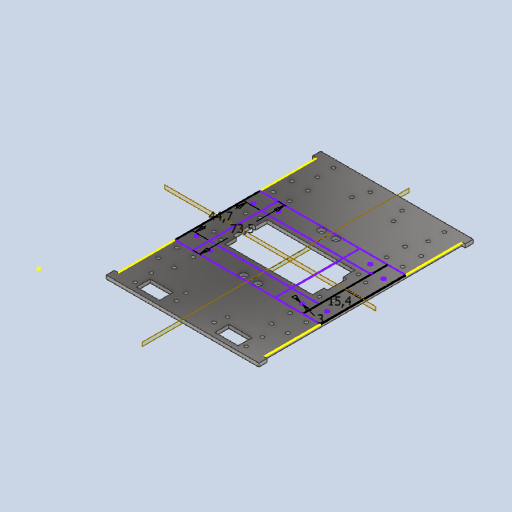
# Autodesk Inventor part: maze_04
Saved by Autodesk Inventor 2022 (Build 260153000, 153)
## iProperties
Created: 2022-07-14
Part Number: maze_04
Material: Сталь нержавеющая, 440C
Document SubType Name: Modeling
Designer: akapu
Density: 7.75 g/cm^3
Appearance: Сталь — полированная
Author: akapu
Autodesk Inventor part; units mm, degrees
ref_plane "YZ Plane" through (0, 0, 0) normal (1, 0, 0) x (0, 1, 0)
ref_plane "XZ Plane" through (0, 0, 0) normal (0, 1, 0) x (-1, 0, 0)
ref_plane "XY Plane" through (0, 0, 0) normal (0, 0, 1) x (1, 0, 0)
sketch "Эскиз2" plane through (0, 0, 0) normal (0, 1, 0) x (-1, 0, 0)
  line L0 (-37, -102) -> (-37, -192)
  line L1 (-166, -192) -> (-163, -192)
  line L2 (-163, -192) -> (-163, -102)
  line L3 (-37, -192) -> (-34, -192)
  line L4 (-34, -200) -> (-166, -200)
  line L5 (-37, -98) -> (-37, -102)
  line L6 (-163, -98) -> (-163, -102)
  line L7 (-166, -192) -> (-166, -200)
  line L8 (-34, -192) -> (-34, -200)
  line L9 (-163, -192) -> (-163, -157)
  line L10 (-163, -157) -> (-37, -157)
  line L11 (-163, -157) -> (-163, -63)
  line L12 (-163, -63) -> (-37, -63)
  line L13 (-34, -34.5) -> (-166, -34.5)
  line L14 (-166, -34.5) -> (-163, -34.5)
  line L15 (-163, -42.5) -> (-166, -42.5)
  line L16 (-166, -42.5) -> (-166, -34.5)
  line L17 (-34, -34.5) -> (-37, -34.5)
  line L18 (-37, -42.5) -> (-34, -42.5)
  line L19 (-37, -98) -> (-37, -34.5)
  line L20 (-34, -34.5) -> (-34, -42.5)
  line L21 (-163, -63) -> (-163, -34.5)
  line L22 (-34, -34.5) -> (-166, -34.5)
  line L23 (-166, -34.5) -> (-166, -24.5)
  line L24 (-166, -24.5) -> (-34, -24.5)
  line L25 (-34, -24.5) -> (-34, -34.5)
  line L26 (-166, -24.5) -> (-34, -24.5)
  line L27 (-34, -24.5) -> (-34, -32.5)
  line L28 (-34, -32.5) -> (-166, -32.5)
  line L29 (-166, -32.5) -> (-166, -24.5)
  line L30 (-34, -32.5) -> (-37, -32.5)
  line L31 (-37, -32.5) -> (-37, -42.5)
  line L32 (-37, -42.5) -> (-34, -42.5)
  line L33 (-34, -42.5) -> (-34, -32.5)
  line L34 (-166, -32.5) -> (-163, -32.5)
  line L35 (-163, -32.5) -> (-163, -42.5)
  line L36 (-163, -42.5) -> (-166, -42.5)
  line L37 (-166, -42.5) -> (-166, -32.5)
  line L38 (-166, -200) -> (-34, -200)
  line L39 (-34, -200) -> (-34, -210)
  line L40 (-34, -210) -> (-166, -210)
  line L41 (-166, -210) -> (-166, -200)
  line L42 (-34, -210) -> (-166, -210)
  line L43 (-166, -210) -> (-166, -202)
  line L44 (-166, -202) -> (-34, -202)
  line L45 (-34, -202) -> (-34, -210)
  line L46 (-163, -192) -> (-166, -192)
  line L47 (-166, -192) -> (-166, -202)
  line L48 (-166, -202) -> (-163, -202)
  line L49 (-163, -202) -> (-163, -192)
  line L50 (-37, -192) -> (-34, -192)
  line L51 (-34, -192) -> (-34, -202)
  line L52 (-34, -202) -> (-37, -202)
  line L53 (-37, -202) -> (-37, -192)
  point P0 (-37, -63)
  dimension "d181" = 94
  dimension "d247" = 8
  dimension "d367" = 10
  dimension "d368" = 8
  dimension "d369" = 10
  dimension "d370" = 8
  constraints: 108 end point, 21 parallel, 11 horizontal, 11 perpendicular, 7 point on line, 3 vertical
  measures "d181" distance of L9.end L11.end
  measures "d247" distance of L14.end L15.start
  measures "d367" distance of L22.end L23.end
  measures "d368" distance of L26.end L27.end
  measures "d369" distance of L38.end L39.end
  measures "d370" distance of L42.end L43.end
extrude "Выдавливание1" add sketch "Эскиз2" along normal blind 3 contours L0 L10 L2 L6 L11 L12 L19 L5 | L0 L53 L4 L49 L2 L10 | L12 L21 L13 L19 | L53 L44 L49 L4 | L44 L39 L40 L41 | L13 L35 L28 L31 | L28 L23 L24 L25
sketch "Эскиз3" plane through (0, 3, 0) normal (0, 1, 0) x (1, 0, 0)
  line L0 (163, 42.5) -> (163, 34.5)
  line L1 (34, 34.5) -> (166, 34.5)
  line L2 (44, 159) -> (58, 159)
  line L3 (58, 159) -> (58, 175)
  line L4 (58, 175) -> (44, 175)
  line L5 (44, 175) -> (44, 159)
  line L6 (142, 159) -> (156, 159)
  line L7 (156, 159) -> (156, 175)
  line L8 (156, 175) -> (142, 175)
  line L9 (142, 175) -> (142, 159)
  line L10 (142, 75.5) -> (156, 75.5)
  line L11 (156, 75.5) -> (156, 59.5)
  line L12 (156, 59.5) -> (142, 59.5)
  line L13 (142, 59.5) -> (142, 75.5)
  line L14 (44, 75.5) -> (58, 75.5)
  line L15 (58, 75.5) -> (58, 59.5)
  line L16 (58, 59.5) -> (44, 59.5)
  line L17 (44, 59.5) -> (44, 75.5)
  circle A0 centre (58, 59.5) radius 1.6
  circle A1 centre (44, 59.5) radius 1.6
  circle A2 centre (44, 75.5) radius 1.6
  circle A3 centre (58, 75.5) radius 1.6
  circle A4 centre (142, 59.5) radius 1.6
  circle A5 centre (156, 59.5) radius 1.6
  circle A6 centre (156, 75.5) radius 1.6
  circle A7 centre (142, 75.5) radius 1.6
  circle A8 centre (156, 175) radius 1.6
  circle A9 centre (156, 159) radius 1.6
  circle A10 centre (142, 159) radius 1.6
  circle A11 centre (142, 175) radius 1.6
  circle A12 centre (58, 175) radius 1.6
  circle A13 centre (58, 159) radius 1.6
  circle A14 centre (44, 159) radius 1.6
  circle A15 centre (44, 175) radius 1.6
  point P0 (0, 0)
  point P1 (37, 63)
  point P2 (37, 42.5)
  dimension "d372" = 16
  dimension "d375" = 16
  dimension "d376" = 3.2
  dimension "d377" = 3.2
  dimension "d378" = 3.2
  dimension "d379" = 3.2
  dimension "d380" = 3.2
  dimension "d381" = 3.2
  dimension "d382" = 3.2
  dimension "d383" = 3.2
  dimension "d384" = 3.2
  dimension "d385" = 3.2
  dimension "d386" = 3.2
  dimension "d387" = 3.2
  dimension "d388" = 3.2
  dimension "d389" = 3.2
  dimension "d390" = 3.2
  dimension "d391" = 3.2
  constraints: 36 end point, 16 centre point, 16 coincident, 3 point on line
  measures "d372" distance of L3.end L2.end
  measures "d375" distance of L10.end L11.end
  measures "d376" diameter of A0
  measures "d377" diameter of A1
  measures "d378" diameter of A2
  measures "d379" diameter of A3
  measures "d380" diameter of A4
  measures "d381" diameter of A5
  measures "d382" diameter of A6
  measures "d383" diameter of A7
  measures "d384" diameter of A8
  measures "d385" diameter of A9
  measures "d386" diameter of A10
  measures "d387" diameter of A11
  measures "d388" diameter of A12
  measures "d389" diameter of A13
  measures "d390" diameter of A14
  measures "d391" diameter of A15
extrude "Выдавливание2" cut sketch "Эскиз3" against normal blind 5 contours L5 A14 L2 | L2 A14 L5 | A13 L3 L2 | L2 L3 A13 | A15 L4 L5 | L5 L4 A15 | A12 L4 L3 | L3 L4 A12 | L9 A10 L6 | L6 A10 L9 | A9 L7 L6 | L6 L7 A9 | A11 L8 L9 | L9 L8 A11 | A8 L8 L7 | L7 L8 A8 | L13 A7 L10 | L10 A7 L13 | A6 L11 L10 | L10 L11 A6 | A4 L12 L13 | L13 L12 A4 | A5 L12 L11 | L11 L12 A5 | L17 A2 L14 | L14 A2 L17 | A3 L15 L14 | L14 L15 A3 | A1 L16 L17 | L17 L16 A1 | A0 L16 L15 | L15 L16 A0
sketch "Эскиз12" plane through (0, 0, 0) normal (0, -1, 0) x (1, 0, 0)
  line L0 (37, -202) -> (37, -32.5) projected
  line L1 (93.8, -83.5) -> (106.2, -83.5)
  line L2 (106.2, -151) -> (93.8, -151)
  circle A0 centre (93.8, -83.5) radius 3
  circle A1 centre (106.2, -83.5) radius 3
  circle A2 centre (106.2, -151) radius 3
  circle A3 centre (93.8, -151) radius 3
  line L3 (137.6, -98.9) -> (137.6, -135.6)
  line L4 (62.4, -135.6) -> (62.4, -98.9)
  line L5 (62.4, -98.9) -> (137.6, -98.9)
  line L6 (137.6, -98.9) -> (137.6, -135.6)
  line L7 (137.6, -135.6) -> (62.4, -135.6)
  line L8 (62.4, -135.6) -> (62.4, -98.9)
  line L9 (137.6, -135.6) -> (138, -135.6)
  line L10 (138, -135.6) -> (62, -135.6)
  line L11 (62, -135.6) -> (62, -98.9)
  line L12 (62, -98.9) -> (138, -98.9)
  line L13 (138, -98.9) -> (138, -135.6)
  point P0 (0, 0)
  point P1 (37, -192)
  dimension "d394" = 6
  dimension "d395" = 6
  dimension "d396" = 6
  dimension "d397" = 6
  dimension "d422" = 75.2
  dimension "d423" = 0.4
  dimension "d424" = 76
  constraints: 26 end point, 4 centre point, 4 coincident, 4 parallel, 3 horizontal, 2 perpendicular, 1 point on line
  measures "d394" diameter of A0
  measures "d395" diameter of A1
  measures "d396" diameter of A2
  measures "d397" diameter of A3
  measures "d422" distance of L3.end L7.end
  measures "d423" distance of L3.end L9.end
  measures "d424" distance of L11.end L12.end
extrude "Выдавливание9" cut sketch "Эскиз12" against normal blind 5
sketch "Эскиз17" plane through (0, 0, 0) normal (0, -1, 0) x (1, 0, 0)
  line L0 (62.4, -98.9) -> (137.6, -98.9)
  line L1 (62.4, -98.9) -> (62.4, -135.6)
  line L2 (137.6, -98.9) -> (62.4, -98.9)
  line L3 (62.4, -98.9) -> (62.4, -135.6)
  line L4 (62.4, -135.6) -> (137.6, -135.6)
  line L5 (137.6, -135.6) -> (137.6, -98.9)
  line L6 (137.6, -135.6) -> (137.6, -98.9)
  line L7 (137.6, -135.6) -> (142.6, -135.6)
  line L8 (142.6, -135.6) -> (142.6, -134)
  line L9 (137.6, -98.9) -> (142.6, -98.9)
  line L10 (142.6, -98.9) -> (142.6, -100.5)
  line L11 (62.4, -135.6) -> (57.4, -135.6)
  line L12 (57.4, -135.6) -> (57.4, -134)
  line L13 (62.4, -98.9) -> (57.4, -98.9)
  line L14 (57.4, -98.9) -> (57.4, -100.5)
  circle A0 centre (142.6, -100.5) radius 1.5
  circle A1 centre (142.6, -134) radius 1.5
  circle A2 centre (57.4, -100.5) radius 1.5
  circle A3 centre (57.4, -134) radius 1.5
  point P0 (0, 0)
  dimension "d432" = 3
  dimension "d407" = 75.2
  dimension "d408" = 36.7
  dimension "d409" = 5
  dimension "d410" = 1.6
  dimension "d411" = 5
  dimension "d412" = 1.6
  dimension "d413" = 5
  dimension "d414" = 1.6
  dimension "d415" = 1.6
  dimension "d416" = 3
  dimension "d417" = 3
  dimension "d418" = 3
  dimension "d419" = 3
  constraints: 30 end point, 4 centre point, 4 coincident
  measures "d407" distance of L1.end L4.end
  measures "d408" distance of L4.end L0.end
  measures "d409" distance of L4.end L7.end
  measures "d410" distance of L7.end L8.end
  measures "d411" distance of L0.end L9.end
  measures "d412" distance of L9.end L10.end
  measures "d413" distance of L1.end L11.end
  measures "d414" distance of L11.end L12.end
  measures "d415" distance of L13.end L14.end
  measures "d416" diameter of A0
  measures "d417" diameter of A1
  measures "d418" diameter of A2
  measures "d419" diameter of A3
extrude "Выдавливание14" cut sketch "Эскиз17" against normal blind 5 contours A0 | A1 | A3 | A2
sketch "Эскиз19" plane through (0, 0, 0) normal (0, -1, 0) x (1, 0, 0)
  line L0 (62, -135.6) -> (62, -98.9) projected
  line L1 (62, -98.9) -> (62, -108.9)
  line L2 (62, -135.6) -> (62, -125.6)
  line L3 (62, -108.9) -> (59, -108.9)
  line L4 (59, -108.9) -> (59, -125.6)
  line L5 (59, -125.6) -> (62, -125.6)
  line L6 (62, -125.6) -> (62, -108.9)
  line L7 (59, -108.9) -> (141, -108.9)
  line L8 (141, -108.9) -> (141, -125.6)
  line L9 (141, -125.6) -> (59, -125.6)
  line L10 (59, -125.6) -> (59, -108.9)
  point P0 (0, 0)
  dimension "d425" = 10
  dimension "d426" = 10
  dimension "d427" = 3
  dimension "d428" = 82
  constraints: 20 end point, 4 parallel, 3 point on line, 2 horizontal, 2 perpendicular
  measures "d425" distance of L0.end L1.end
  measures "d426" distance of L0.start L2.end
  measures "d427" distance of L5.end L4.end
  measures "d428" distance of L8.end L9.end
extrude "Выдавливание15" cut sketch "Эскиз19" against normal blind 5
sketch "Эскиз20" plane through (0, 3, 0) normal (0, 1, 0) x (1, 0, 0)
  line L0 (37, 202) -> (37, 32.5) projected
  line L1 (34, 32.5) -> (34, 24.5) projected
  line L2 (37, 32.5) -> (34, 32.5)
  line L3 (34, 32.5) -> (34, 31.5)
  line L4 (34, 31.5) -> (37, 31.5)
  line L5 (37, 31.5) -> (37, 32.5)
  line L6 (34, 210) -> (34, 202) projected
  line L7 (34, 202) -> (37, 202)
  line L8 (37, 202) -> (37, 203)
  line L9 (37, 203) -> (34, 203)
  line L10 (34, 203) -> (34, 202)
  line L11 (163, 32.5) -> (163, 202) projected
  line L12 (166, 202) -> (166, 210) projected
  line L13 (163, 202) -> (166, 202)
  line L14 (166, 202) -> (166, 203)
  line L15 (166, 203) -> (163, 203)
  line L16 (163, 203) -> (163, 202)
  line L17 (166, 24.5) -> (166, 32.5) projected
  line L18 (163, 32.5) -> (166, 32.5)
  line L19 (166, 32.5) -> (166, 31.5)
  line L20 (166, 31.5) -> (163, 31.5)
  line L21 (163, 31.5) -> (163, 32.5)
  point P0 (0, 0)
  dimension "d431" = 1
  dimension "d432" = 3
  dimension "d433" = 1
  constraints: 32 end point, 8 parallel, 7 point on line, 4 horizontal, 4 perpendicular
  measures "d431" distance of L3.end L2.end
  measures "d432" distance of L9.end L8.end
  measures "d433" distance of L8.end L7.end
extrude "Выдавливание16" cut sketch "Эскиз20" against normal blind 10
sketch "Эскиз21" plane through (0, 3, 0) normal (0, 1, 0) x (1, 0, 0)
  line L0 (34, 24.5) -> (166, 24.5) projected
  line L1 (166, 24.5) -> (166, 31.5) projected
  line L2 (166, 24.5) -> (166, 31.5)
  line L3 (34, 31.5) -> (34, 24.5) projected
  line L4 (166, 31.5) -> (34, 31.5)
  line L5 (34, 31.5) -> (34, 45.5)
  line L6 (34, 45.5) -> (163, 45.5)
  line L7 (163, 203) -> (163, 31.5) projected
  line L8 (166, 210) -> (34, 210) projected
  line L9 (34, 210) -> (34, 203) projected
  line L10 (34, 210) -> (34, 203)
  line L11 (34, 203) -> (166, 203)
  line L12 (37, 203) -> (37, 31.5) projected
  line L13 (37, 203) -> (52, 203)
  line L14 (52, 203) -> (82, 203)
  line L15 (163, 203) -> (148, 203)
  line L16 (148, 203) -> (118, 203)
  circle A0 centre (52, 203) radius 1.5
  circle A1 centre (82, 203) radius 1.5
  circle A2 centre (118, 203) radius 1.5
  circle A3 centre (148, 203) radius 1.5
  circle A4 centre (148, 45.5) radius 1.5
  circle A5 centre (148, 31.5) radius 1.5
  circle A6 centre (118, 31.5) radius 1.5
  circle A7 centre (118, 45.5) radius 1.5
  circle A8 centre (82, 45.5) radius 1.5
  circle A9 centre (82, 31.5) radius 1.5
  circle A10 centre (52, 45.5) radius 1.5
  circle A11 centre (52, 31.5) radius 1.5
  line L17 (163, 203) -> (163, 189)
  line L18 (163, 189) -> (37, 189)
  circle A12 centre (52, 189) radius 1.5
  circle A13 centre (82, 189) radius 1.5
  circle A14 centre (118, 189) radius 1.5
  circle A15 centre (148, 189) radius 1.5
  circle A16 centre (113.75, 200.62) radius 1.5 projected
  circle A17 centre (86.25, 200.62) radius 1.5 projected
  circle A18 centre (52, 203.03) radius 1.5 projected
  circle A19 centre (52, 31.5) radius 1.5 projected
  circle A20 centre (52, 45.5) radius 1.5 projected
  circle A21 centre (82, 45.5) radius 1.5 projected
  circle A22 centre (82, 189.03) radius 1.5 projected
  circle A23 centre (52, 189.03) radius 1.5 projected
  circle A24 centre (148, 31.5) radius 1.5 projected
  circle A25 centre (118, 189.03) radius 1.5 projected
  circle A26 centre (148, 189.03) radius 1.5 projected
  circle A27 centre (118, 45.5) radius 1.5 projected
  circle A28 centre (148, 203.03) radius 1.5 projected
  circle A29 centre (148, 45.5) radius 1.5 projected
  arc A30 (163, 49.5) -> (160, 52.5) centre (160, 49.5) ccw projected
  line L19 (163, 49.5) -> (163, 31.5) projected
  line L20 (163, 31.5) -> (180, 31.5) projected
  arc A31 (180, 31.5) -> (183, 34.5) centre (180, 34.5) ccw projected
  line L21 (183, 34.5) -> (183, 200.03) projected
  arc A32 (183, 200.03) -> (180, 203.03) centre (180, 200.03) ccw projected
  line L22 (163, 203.03) -> (180, 203.03) projected
  line L23 (163, 203.03) -> (163, 185.03) projected
  arc A33 (160, 182.03) -> (163, 185.03) centre (160, 185.03) ccw projected
  line L24 (160, 182.03) -> (40, 182.03) projected
  arc A34 (37, 185.03) -> (40, 182.03) centre (40, 185.03) ccw projected
  line L25 (37, 185.03) -> (37, 203.03) projected
  line L26 (37, 203.03) -> (20, 203.03) projected
  arc A35 (20, 203.03) -> (17, 200.03) centre (20, 200.03) ccw projected
  line L27 (17, 200.03) -> (17, 34.5) projected
  arc A36 (17, 34.5) -> (20, 31.5) centre (20, 34.5) ccw projected
  line L28 (37, 31.5) -> (20, 31.5) projected
  line L29 (37, 31.5) -> (37, 49.5) projected
  arc A37 (40, 52.5) -> (37, 49.5) centre (40, 49.5) ccw projected
  line L30 (40, 52.5) -> (160, 52.5) projected
  line L31 (174.5, 24.5) -> (25.5, 24.5) projected
  spline S0 degree 3 poles (11, 35.5558) (11.7825, 25.694) (15.7005, 25.8128) (25.5, 24.5) knots -0.786777 -0.786777 -0.786777 -0.786777 0 0 0 0 projected
  line L32 (11, 198.9742) -> (11, 35.5558) projected
  line L33 (189, 35.5558) -> (189, 198.9742) projected
  spline S1 degree 3 poles (189, 35.5558) (188.2175, 25.694) (184.2995, 25.8128) (174.5, 24.5) knots -0.786777 -0.786777 -0.786777 -0.786777 0 0 0 0 projected
  circle A38 centre (83.77, 35.5) radius 1.6 projected
  line L34 (123.978, 28.5) -> (143, 28.5) projected
  line L35 (143, 28.5) -> (143, 40.5) projected
  line L36 (143, 40.5) -> (123.978, 40.5) projected
  line L37 (123.978, 40.5) -> (123.978, 28.5) projected
  circle A39 centre (116.23, 35.5) radius 1.6 projected
  line L38 (57, 28.5) -> (76.022, 28.5) projected
  line L39 (76.022, 28.5) -> (76.022, 40.5) projected
  line L40 (76.022, 40.5) -> (57, 40.5) projected
  line L41 (57, 40.5) -> (57, 28.5) projected
  circle A40 centre (113.75, 200.62) radius 1.5 projected
  circle A41 centre (86.25, 200.62) radius 1.5 projected
  circle A42 centre (52, 203.03) radius 1.5 projected
  circle A43 centre (52, 31.5) radius 1.5 projected
  circle A44 centre (52, 45.5) radius 1.5 projected
  circle A45 centre (82, 45.5) radius 1.5 projected
  circle A46 centre (82, 189.03) radius 1.5 projected
  circle A47 centre (52, 189.03) radius 1.5 projected
  circle A48 centre (148, 31.5) radius 1.5 projected
  circle A49 centre (118, 189.03) radius 1.5 projected
  circle A50 centre (148, 189.03) radius 1.5 projected
  circle A51 centre (118, 45.5) radius 1.5 projected
  circle A52 centre (148, 203.03) radius 1.5 projected
  circle A53 centre (148, 45.5) radius 1.5 projected
  arc A54 (163, 49.5) -> (160, 52.5) centre (160, 49.5) ccw projected
  line L42 (163, 49.5) -> (163, 31.5) projected
  line L43 (163, 31.5) -> (180, 31.5) projected
  arc A55 (180, 31.5) -> (183, 34.5) centre (180, 34.5) ccw projected
  line L44 (183, 34.5) -> (183, 200.03) projected
  arc A56 (183, 200.03) -> (180, 203.03) centre (180, 200.03) ccw projected
  line L45 (163, 203.03) -> (180, 203.03) projected
  line L46 (163, 203.03) -> (163, 185.03) projected
  arc A57 (160, 182.03) -> (163, 185.03) centre (160, 185.03) ccw projected
  line L47 (160, 182.03) -> (40, 182.03) projected
  arc A58 (37, 185.03) -> (40, 182.03) centre (40, 185.03) ccw projected
  line L48 (37, 185.03) -> (37, 203.03) projected
  line L49 (37, 203.03) -> (20, 203.03) projected
  arc A59 (20, 203.03) -> (17, 200.03) centre (20, 200.03) ccw projected
  line L50 (17, 200.03) -> (17, 34.5) projected
  arc A60 (17, 34.5) -> (20, 31.5) centre (20, 34.5) ccw projected
  line L51 (37, 31.5) -> (20, 31.5) projected
  line L52 (37, 31.5) -> (37, 49.5) projected
  arc A61 (40, 52.5) -> (37, 49.5) centre (40, 49.5) ccw projected
  line L53 (40, 52.5) -> (160, 52.5) projected
  line L54 (174.5, 24.5) -> (25.5, 24.5) projected
  spline S2 degree 3 poles (11, 35.5558) (11.7825, 25.694) (15.7005, 25.8128) (25.5, 24.5) knots -0.786777 -0.786777 -0.786777 -0.786777 0 0 0 0 projected
  line L55 (11, 198.9742) -> (11, 35.5558) projected
  line L56 (189, 35.5558) -> (189, 198.9742) projected
  spline S3 degree 3 poles (189, 35.5558) (188.2175, 25.694) (184.2995, 25.8128) (174.5, 24.5) knots -0.786777 -0.786777 -0.786777 -0.786777 0 0 0 0 projected
  circle A62 centre (83.77, 35.5) radius 1.6 projected
  line L57 (123.978, 28.5) -> (143, 28.5) projected
  line L58 (143, 28.5) -> (143, 40.5) projected
  line L59 (143, 40.5) -> (123.978, 40.5) projected
  line L60 (123.978, 40.5) -> (123.978, 28.5) projected
  circle A63 centre (116.23, 35.5) radius 1.6 projected
  line L61 (57, 28.5) -> (76.022, 28.5) projected
  line L62 (76.022, 28.5) -> (76.022, 40.5) projected
  line L63 (76.022, 40.5) -> (57, 40.5) projected
  line L64 (57, 40.5) -> (57, 28.5) projected
  circle A64 centre (113.75, 200.62) radius 1.5 projected
  circle A65 centre (86.25, 200.62) radius 1.5 projected
  circle A66 centre (52, 203.03) radius 1.5 projected
  circle A67 centre (52, 31.5) radius 1.5 projected
  circle A68 centre (52, 45.5) radius 1.5 projected
  circle A69 centre (82, 45.5) radius 1.5 projected
  circle A70 centre (82, 189.03) radius 1.5 projected
  circle A71 centre (52, 189.03) radius 1.5 projected
  circle A72 centre (148, 31.5) radius 1.5 projected
  circle A73 centre (118, 189.03) radius 1.5 projected
  circle A74 centre (148, 189.03) radius 1.5 projected
  circle A75 centre (118, 45.5) radius 1.5 projected
  circle A76 centre (148, 203.03) radius 1.5 projected
  circle A77 centre (148, 45.5) radius 1.5 projected
  arc A78 (163, 49.5) -> (160, 52.5) centre (160, 49.5) ccw projected
  line L65 (163, 49.5) -> (163, 31.5) projected
  line L66 (163, 31.5) -> (180, 31.5) projected
  arc A79 (180, 31.5) -> (183, 34.5) centre (180, 34.5) ccw projected
  line L67 (183, 34.5) -> (183, 200.03) projected
  arc A80 (183, 200.03) -> (180, 203.03) centre (180, 200.03) ccw projected
  line L68 (163, 203.03) -> (180, 203.03) projected
  line L69 (163, 203.03) -> (163, 185.03) projected
  arc A81 (160, 182.03) -> (163, 185.03) centre (160, 185.03) ccw projected
  line L70 (160, 182.03) -> (40, 182.03) projected
  arc A82 (37, 185.03) -> (40, 182.03) centre (40, 185.03) ccw projected
  line L71 (37, 185.03) -> (37, 203.03) projected
  line L72 (37, 203.03) -> (20, 203.03) projected
  arc A83 (20, 203.03) -> (17, 200.03) centre (20, 200.03) ccw projected
  line L73 (17, 200.03) -> (17, 34.5) projected
  arc A84 (17, 34.5) -> (20, 31.5) centre (20, 34.5) ccw projected
  line L74 (37, 31.5) -> (20, 31.5) projected
  line L75 (37, 31.5) -> (37, 49.5) projected
  arc A85 (40, 52.5) -> (37, 49.5) centre (40, 49.5) ccw projected
  line L76 (40, 52.5) -> (160, 52.5) projected
  line L77 (174.5, 24.5) -> (25.5, 24.5) projected
  spline S4 degree 3 poles (11, 35.5558) (11.7825, 25.694) (15.7005, 25.8128) (25.5, 24.5) knots -0.786777 -0.786777 -0.786777 -0.786777 0 0 0 0 projected
  line L78 (11, 198.9742) -> (11, 35.5558) projected
  line L79 (189, 35.5558) -> (189, 198.9742) projected
  spline S5 degree 3 poles (189, 35.5558) (188.2175, 25.694) (184.2995, 25.8128) (174.5, 24.5) knots -0.786777 -0.786777 -0.786777 -0.786777 0 0 0 0 projected
  circle A86 centre (83.77, 35.5) radius 1.6 projected
  line L80 (123.978, 28.5) -> (143, 28.5) projected
  line L81 (143, 28.5) -> (143, 40.5) projected
  line L82 (143, 40.5) -> (123.978, 40.5) projected
  line L83 (123.978, 40.5) -> (123.978, 28.5) projected
  circle A87 centre (116.23, 35.5) radius 1.6 projected
  line L84 (57, 28.5) -> (76.022, 28.5) projected
  line L85 (76.022, 28.5) -> (76.022, 40.5) projected
  line L86 (76.022, 40.5) -> (57, 40.5) projected
  line L87 (57, 40.5) -> (57, 28.5) projected
  circle A88 centre (113.75, 200.62) radius 1.5 projected
  circle A89 centre (86.25, 200.62) radius 1.5 projected
  circle A90 centre (52, 203.03) radius 1.5 projected
  circle A91 centre (52, 31.5) radius 1.5 projected
  circle A92 centre (52, 45.5) radius 1.5 projected
  circle A93 centre (82, 45.5) radius 1.5 projected
  circle A94 centre (82, 189.03) radius 1.5 projected
  circle A95 centre (52, 189.03) radius 1.5 projected
  circle A96 centre (148, 31.5) radius 1.5 projected
  circle A97 centre (118, 189.03) radius 1.5 projected
  circle A98 centre (148, 189.03) radius 1.5 projected
  circle A99 centre (118, 45.5) radius 1.5 projected
  circle A100 centre (148, 203.03) radius 1.5 projected
  circle A101 centre (148, 45.5) radius 1.5 projected
  arc A102 (163, 49.5) -> (160, 52.5) centre (160, 49.5) ccw projected
  line L88 (163, 49.5) -> (163, 31.5) projected
  line L89 (163, 31.5) -> (180, 31.5) projected
  arc A103 (180, 31.5) -> (183, 34.5) centre (180, 34.5) ccw projected
  line L90 (183, 34.5) -> (183, 200.03) projected
  arc A104 (183, 200.03) -> (180, 203.03) centre (180, 200.03) ccw projected
  line L91 (163, 203.03) -> (180, 203.03) projected
  line L92 (163, 203.03) -> (163, 185.03) projected
  arc A105 (160, 182.03) -> (163, 185.03) centre (160, 185.03) ccw projected
  line L93 (160, 182.03) -> (40, 182.03) projected
  arc A106 (37, 185.03) -> (40, 182.03) centre (40, 185.03) ccw projected
  line L94 (37, 185.03) -> (37, 203.03) projected
  line L95 (37, 203.03) -> (20, 203.03) projected
  arc A107 (20, 203.03) -> (17, 200.03) centre (20, 200.03) ccw projected
  line L96 (17, 200.03) -> (17, 34.5) projected
  arc A108 (17, 34.5) -> (20, 31.5) centre (20, 34.5) ccw projected
  line L97 (37, 31.5) -> (20, 31.5) projected
  line L98 (37, 31.5) -> (37, 49.5) projected
  arc A109 (40, 52.5) -> (37, 49.5) centre (40, 49.5) ccw projected
  line L99 (40, 52.5) -> (160, 52.5) projected
  line L100 (174.5, 24.5) -> (25.5, 24.5) projected
  spline S6 degree 3 poles (11, 35.5558) (11.7825, 25.694) (15.7005, 25.8128) (25.5, 24.5) knots -0.786777 -0.786777 -0.786777 -0.786777 0 0 0 0 projected
  line L101 (11, 198.9742) -> (11, 35.5558) projected
  line L102 (189, 35.5558) -> (189, 198.9742) projected
  spline S7 degree 3 poles (189, 35.5558) (188.2175, 25.694) (184.2995, 25.8128) (174.5, 24.5) knots -0.786777 -0.786777 -0.786777 -0.786777 0 0 0 0 projected
  circle A110 centre (83.77, 35.5) radius 1.6 projected
  line L103 (123.978, 28.5) -> (143, 28.5) projected
  line L104 (143, 28.5) -> (143, 40.5) projected
  line L105 (143, 40.5) -> (123.978, 40.5) projected
  line L106 (123.978, 40.5) -> (123.978, 28.5) projected
  circle A111 centre (116.23, 35.5) radius 1.6 projected
  line L107 (57, 28.5) -> (76.022, 28.5) projected
  line L108 (76.022, 28.5) -> (76.022, 40.5) projected
  line L109 (76.022, 40.5) -> (57, 40.5) projected
  line L110 (57, 40.5) -> (57, 28.5) projected
  circle A112 centre (113.75, 200.62) radius 1.5 projected
  circle A113 centre (86.25, 200.62) radius 1.5 projected
  circle A114 centre (52, 203.03) radius 1.5 projected
  circle A115 centre (52, 31.5) radius 1.5 projected
  circle A116 centre (52, 45.5) radius 1.5 projected
  circle A117 centre (82, 45.5) radius 1.5 projected
  circle A118 centre (82, 189.03) radius 1.5 projected
  circle A119 centre (52, 189.03) radius 1.5 projected
  circle A120 centre (148, 31.5) radius 1.5 projected
  circle A121 centre (118, 189.03) radius 1.5 projected
  circle A122 centre (148, 189.03) radius 1.5 projected
  circle A123 centre (118, 45.5) radius 1.5 projected
  circle A124 centre (148, 203.03) radius 1.5 projected
  circle A125 centre (148, 45.5) radius 1.5 projected
  arc A126 (163, 49.5) -> (160, 52.5) centre (160, 49.5) ccw projected
  line L111 (163, 49.5) -> (163, 31.5) projected
  line L112 (163, 31.5) -> (180, 31.5) projected
  arc A127 (180, 31.5) -> (183, 34.5) centre (180, 34.5) ccw projected
  line L113 (183, 34.5) -> (183, 200.03) projected
  arc A128 (183, 200.03) -> (180, 203.03) centre (180, 200.03) ccw projected
  line L114 (163, 203.03) -> (180, 203.03) projected
  line L115 (163, 203.03) -> (163, 185.03) projected
  arc A129 (160, 182.03) -> (163, 185.03) centre (160, 185.03) ccw projected
  line L116 (160, 182.03) -> (40, 182.03) projected
  arc A130 (37, 185.03) -> (40, 182.03) centre (40, 185.03) ccw projected
  line L117 (37, 185.03) -> (37, 203.03) projected
  line L118 (37, 203.03) -> (20, 203.03) projected
  arc A131 (20, 203.03) -> (17, 200.03) centre (20, 200.03) ccw projected
  line L119 (17, 200.03) -> (17, 34.5) projected
  arc A132 (17, 34.5) -> (20, 31.5) centre (20, 34.5) ccw projected
  line L120 (37, 31.5) -> (20, 31.5) projected
  line L121 (37, 31.5) -> (37, 49.5) projected
  arc A133 (40, 52.5) -> (37, 49.5) centre (40, 49.5) ccw projected
  line L122 (40, 52.5) -> (160, 52.5) projected
  line L123 (174.5, 24.5) -> (25.5, 24.5) projected
  spline S8 degree 3 poles (11, 35.5558) (11.7825, 25.694) (15.7005, 25.8128) (25.5, 24.5) knots -0.786777 -0.786777 -0.786777 -0.786777 0 0 0 0 projected
  line L124 (11, 198.9742) -> (11, 35.5558) projected
  line L125 (189, 35.5558) -> (189, 198.9742) projected
  spline S9 degree 3 poles (189, 35.5558) (188.2175, 25.694) (184.2995, 25.8128) (174.5, 24.5) knots -0.786777 -0.786777 -0.786777 -0.786777 0 0 0 0 projected
  circle A134 centre (83.77, 35.5) radius 1.6 projected
  line L126 (123.978, 28.5) -> (143, 28.5) projected
  line L127 (143, 28.5) -> (143, 40.5) projected
  line L128 (143, 40.5) -> (123.978, 40.5) projected
  line L129 (123.978, 40.5) -> (123.978, 28.5) projected
  circle A135 centre (116.23, 35.5) radius 1.6 projected
  line L130 (57, 28.5) -> (76.022, 28.5) projected
  line L131 (76.022, 28.5) -> (76.022, 40.5) projected
  line L132 (76.022, 40.5) -> (57, 40.5) projected
  line L133 (57, 40.5) -> (57, 28.5) projected
  circle A136 centre (113.75, 200.62) radius 1.5 projected
  circle A137 centre (86.25, 200.62) radius 1.5 projected
  circle A138 centre (52, 203.03) radius 1.5 projected
  circle A139 centre (52, 31.5) radius 1.5 projected
  circle A140 centre (52, 45.5) radius 1.5 projected
  circle A141 centre (82, 45.5) radius 1.5 projected
  circle A142 centre (82, 189.03) radius 1.5 projected
  circle A143 centre (52, 189.03) radius 1.5 projected
  circle A144 centre (148, 31.5) radius 1.5 projected
  circle A145 centre (118, 189.03) radius 1.5 projected
  circle A146 centre (148, 189.03) radius 1.5 projected
  circle A147 centre (118, 45.5) radius 1.5 projected
  circle A148 centre (148, 203.03) radius 1.5 projected
  circle A149 centre (148, 45.5) radius 1.5 projected
  arc A150 (163, 49.5) -> (160, 52.5) centre (160, 49.5) ccw projected
  line L134 (163, 49.5) -> (163, 31.5) projected
  line L135 (163, 31.5) -> (180, 31.5) projected
  arc A151 (180, 31.5) -> (183, 34.5) centre (180, 34.5) ccw projected
  line L136 (183, 34.5) -> (183, 200.03) projected
  arc A152 (183, 200.03) -> (180, 203.03) centre (180, 200.03) ccw projected
  line L137 (163, 203.03) -> (180, 203.03) projected
  line L138 (163, 203.03) -> (163, 185.03) projected
  arc A153 (160, 182.03) -> (163, 185.03) centre (160, 185.03) ccw projected
  line L139 (160, 182.03) -> (40, 182.03) projected
  arc A154 (37, 185.03) -> (40, 182.03) centre (40, 185.03) ccw projected
  line L140 (37, 185.03) -> (37, 203.03) projected
  line L141 (37, 203.03) -> (20, 203.03) projected
  arc A155 (20, 203.03) -> (17, 200.03) centre (20, 200.03) ccw projected
  line L142 (17, 200.03) -> (17, 34.5) projected
  arc A156 (17, 34.5) -> (20, 31.5) centre (20, 34.5) ccw projected
  line L143 (37, 31.5) -> (20, 31.5) projected
  line L144 (37, 31.5) -> (37, 49.5) projected
  arc A157 (40, 52.5) -> (37, 49.5) centre (40, 49.5) ccw projected
  line L145 (40, 52.5) -> (160, 52.5) projected
  line L146 (174.5, 24.5) -> (25.5, 24.5) projected
  spline S10 degree 3 poles (11, 35.5558) (11.7825, 25.694) (15.7005, 25.8128) (25.5, 24.5) knots -0.786777 -0.786777 -0.786777 -0.786777 0 0 0 0 projected
  line L147 (11, 198.9742) -> (11, 35.5558) projected
  line L148 (189, 35.5558) -> (189, 198.9742) projected
  spline S11 degree 3 poles (189, 35.5558) (188.2175, 25.694) (184.2995, 25.8128) (174.5, 24.5) knots -0.786777 -0.786777 -0.786777 -0.786777 0 0 0 0 projected
  circle A158 centre (83.77, 35.5) radius 1.6 projected
  line L149 (123.978, 28.5) -> (143, 28.5) projected
  line L150 (143, 28.5) -> (143, 40.5) projected
  line L151 (143, 40.5) -> (123.978, 40.5) projected
  line L152 (123.978, 40.5) -> (123.978, 28.5) projected
  circle A159 centre (116.23, 35.5) radius 1.6 projected
  line L153 (57, 28.5) -> (76.022, 28.5) projected
  line L154 (76.022, 28.5) -> (76.022, 40.5) projected
  line L155 (76.022, 40.5) -> (57, 40.5) projected
  line L156 (57, 40.5) -> (57, 28.5) projected
  circle A160 centre (86.25, 200.62) radius 1.5 projected
  arc A161 (87.1837, 199.446) -> (84.9779, 201.4149) centre (86.25, 200.62) ccw projected
  arc A162 (87.1837, 199.446) -> (84.9779, 201.4149) centre (86.25, 200.62) ccw projected
  circle A163 centre (86.25, 200.62) radius 1.5
  circle A164 centre (113.75, 200.62) radius 1.5
  spline S12 degree 3 poles (11, 198.9742) (11.7765, 208.7602) (15.6405, 208.7185) (25.2752, 210) knots -0.786777 -0.786777 -0.786777 -0.786777 -0.006043 -0.006043 -0.006043 -0.006043 projected
  spline S13 degree 3 poles (189, 198.9742) (188.2235, 208.7602) (184.3595, 208.7185) (174.7248, 210) knots -0.786777 -0.786777 -0.786777 -0.786777 -0.006043 -0.006043 -0.006043 -0.006043 projected
  line L157 (25.2752, 210) -> (174.7248, 210) projected
  spline S14 degree 3 poles (11, 198.9742) (11.7765, 208.7602) (15.6405, 208.7185) (25.2752, 210) knots -0.786777 -0.786777 -0.786777 -0.786777 -0.006043 -0.006043 -0.006043 -0.006043 projected
  spline S15 degree 3 poles (189, 198.9742) (188.2235, 208.7602) (184.3595, 208.7185) (174.7248, 210) knots -0.786777 -0.786777 -0.786777 -0.786777 -0.006043 -0.006043 -0.006043 -0.006043 projected
  line L158 (25.2752, 210) -> (174.7248, 210) projected
  spline S16 degree 3 poles (11, 198.9742) (11.7765, 208.7602) (15.6405, 208.7185) (25.2752, 210) knots -0.786777 -0.786777 -0.786777 -0.786777 -0.006043 -0.006043 -0.006043 -0.006043 projected
  spline S17 degree 3 poles (189, 198.9742) (188.2235, 208.7602) (184.3595, 208.7185) (174.7248, 210) knots -0.786777 -0.786777 -0.786777 -0.786777 -0.006043 -0.006043 -0.006043 -0.006043 projected
  line L159 (25.2752, 210) -> (174.7248, 210) projected
  spline S18 degree 3 poles (11, 198.9742) (11.7765, 208.7602) (15.6405, 208.7185) (25.2752, 210) knots -0.786777 -0.786777 -0.786777 -0.786777 -0.006043 -0.006043 -0.006043 -0.006043 projected
  spline S19 degree 3 poles (189, 198.9742) (188.2235, 208.7602) (184.3595, 208.7185) (174.7248, 210) knots -0.786777 -0.786777 -0.786777 -0.786777 -0.006043 -0.006043 -0.006043 -0.006043 projected
  line L160 (25.2752, 210) -> (174.7248, 210) projected
  spline S20 degree 3 poles (11, 198.9742) (11.7765, 208.7602) (15.6405, 208.7185) (25.2752, 210) knots -0.786777 -0.786777 -0.786777 -0.786777 -0.006043 -0.006043 -0.006043 -0.006043 projected
  spline S21 degree 3 poles (189, 198.9742) (188.2235, 208.7602) (184.3595, 208.7185) (174.7248, 210) knots -0.786777 -0.786777 -0.786777 -0.786777 -0.006043 -0.006043 -0.006043 -0.006043 projected
  line L161 (25.2752, 210) -> (174.7248, 210) projected
  spline S22 degree 3 poles (11, 198.9742) (11.7765, 208.7602) (15.6405, 208.7185) (25.2752, 210) knots -0.786777 -0.786777 -0.786777 -0.786777 -0.006043 -0.006043 -0.006043 -0.006043 projected
  spline S23 degree 3 poles (189, 198.9742) (188.2235, 208.7602) (184.3595, 208.7185) (174.7248, 210) knots -0.786777 -0.786777 -0.786777 -0.786777 -0.006043 -0.006043 -0.006043 -0.006043 projected
  line L162 (25.2752, 210) -> (174.7248, 210) projected
  point P0 (0, 0)
  point P1 (25.5, 210.03)
  point P2 (174.5, 210.03)
  dimension "d436" = 14
  dimension "d438" = 15
  dimension "d441" = 30
  dimension "d442" = 3
  dimension "d445" = 3
  dimension "d446" = 3
  dimension "d449" = 3
  dimension "d450" = 3
  dimension "d451" = 3
  dimension "d452" = 3
  dimension "d453" = 3
  dimension "d454" = 3
  dimension "d455" = 3
  dimension "d456" = 3
  dimension "d457" = 3
  dimension "d460" = 14
  dimension "d461" = 3
  dimension "d462" = 3
  dimension "d463" = 3
  dimension "d464" = 3
  constraints: 24 end point, 18 centre point, 15 point on line, 6 coincident, 5 perpendicular, 2 concentric, 1 collinear, 1 vertical
  measures "d436" distance of L3.start L5.end
  measures "d438" distance of L12.start L13.end
  measures "d441" distance of L15.end L16.end
  measures "d442" diameter of A0
  measures "d445" diameter of A1
  measures "d446" diameter of A2
  measures "d449" diameter of A3
  measures "d450" diameter of A4
  measures "d451" diameter of A5
  measures "d452" diameter of A6
  measures "d453" diameter of A7
  measures "d454" diameter of A8
  measures "d455" diameter of A9
  measures "d456" diameter of A10
  measures "d457" diameter of A11
  measures "d460" distance of L7.start L17.end
  measures "d461" diameter of A12
  measures "d462" diameter of A13
  measures "d463" diameter of A14
  measures "d464" diameter of A15
extrude "Выдавливание17" cut sketch "Эскиз21" against normal blind 10 contours A11 L4 | L4 A11 | A5 L4 | L4 A5 | A10 L6 | L6 A10 | A4 L6 | L6 A4 | A8 L6 | L6 A8 | A7 L6 | L6 A7 | A12 L18 | A23 A12 | L18 A23 | A26 L18 | L18 A15 | A15 A26 | A0 L11 | A18 A0 | L11 A18 | A28 L11 | L11 A3 | A3 A28 | A13 L18 | A22 A13 | L18 A22 | A25 L18 | L18 A14 | A14 A25 | A16 | A17 picked at (51.9405, 187.5208) picked at (147.9405, 187.5208) picked at (51.9405, 201.5208) picked at (147.9405, 201.5208) picked at (81.9405, 187.5208) picked at (117.9405, 187.5208)
sketch "Эскиз29" plane through (0, 3, 0) normal (0, 1, 0) x (1, 0, 0)
  line L0 (34, 24.5) -> (166, 24.5) projected
  line L1 (100, 24.5) -> (116.227, 24.5)
  line L2 (116.227, 35.5) -> (83.773, 35.5)
  line L3 (83.773, 35.5) -> (76.022, 35.5)
  circle A0 centre (52, 31.5) radius 1.5 projected
  line L4 (58, 31.5) -> (58, 35.5)
  circle A1 centre (148, 31.5) radius 1.5 projected
  line L5 (142, 31.5) -> (142, 35.5)
  line L6 (116.227, 35.5) -> (123.978, 35.5)
  line L7 (76.022, 35.5) -> (76.022, 40.5)
  line L8 (76.022, 40.5) -> (76.022, 28.5)
  line L9 (123.978, 35.5) -> (123.978, 40.5)
  line L10 (123.978, 40.5) -> (123.978, 28.5)
  line L11 (123.978, 28.5) -> (142, 28.5)
  line L12 (142, 28.5) -> (142, 40.5)
  line L13 (142, 40.5) -> (123.978, 40.5)
  line L14 (76.022, 40.5) -> (58, 40.5)
  line L15 (58, 40.5) -> (58, 28.5)
  line L16 (58, 28.5) -> (76.022, 28.5)
  line L17 (100, 24.5) -> (100, 35.5)
  line L18 (100, 35.5) -> (83.77, 35.5)
  line L19 (83.77, 35.5) -> (116.23, 35.5)
  circle A2 centre (83.77, 35.5) radius 1.6
  circle A3 centre (116.23, 35.5) radius 1.6
  point P0 (0, 0)
  dimension "d503" = 16.227
  dimension "d504" = 11
  dimension "d505" = 32.454
  dimension "d510" = 6
  dimension "d511" = 7.751
  dimension "d514" = 5
  dimension "d515" = 12
  dimension "d532" = 32.46
  dimension "d533" = 3.2
  dimension "d534" = 3.2
  constraints: 38 end point, 8 point on line, 4 coincident, 4 perpendicular, 2 centre point, 2 midpoint, 2 vertical, 1 collinear, 1 horizontal
  measures "d503" distance of L1.start L1.end
  measures "d504" distance of L1.end L2.start
  measures "d505" distance of L2.start L2.end
  measures "d510" distance of A1.centre L5.start
  measures "d511" distance of L6.start L6.end
  measures "d514" distance of L3.end L7.end
  measures "d515" distance of L7.end L8.end
  measures "d532" distance of L18.end L19.end
  measures "d533" diameter of A2
  measures "d534" diameter of A3
extrude "Выдавливание21" cut sketch "Эскиз29" against normal blind 3 contours L8 L16 L15 L4 L14 L7 | A2 L3 L2 | L2 L3 A2 | L9 L13 L12 L5 L11 L10 | A3 L6 L2 | L2 L6 A3
sketch "Эскиз30" plane through (0, 3, 0) normal (0, 1, 0) x (1, 0, 0)
  line L0 (76.022, 40.5) -> (58, 40.5) projected
  line L1 (58, 40.5) -> (56, 40.5)
  line L2 (56, 40.5) -> (56, 28.5)
  line L3 (58, 28.5) -> (76.022, 28.5) projected
  line L4 (56, 28.5) -> (58, 28.5)
  line L5 (142, 40.5) -> (123.978, 40.5) projected
  line L6 (142, 40.5) -> (144, 40.5)
  line L7 (144, 40.5) -> (144, 28.5)
  line L8 (144, 28.5) -> (142, 28.5)
  line L9 (142, 28.5) -> (142, 40.5)
  line L10 (58, 40.5) -> (58, 28.5) projected
  line L11 (58, 40.5) -> (58, 28.5)
  point P0 (0, 0)
  dimension "d518" = 2
  dimension "d519" = 2
  constraints: 16 end point, 5 perpendicular, 2 horizontal, 1 collinear
  measures "d518" distance of L0.end L1.end
  measures "d519" distance of L5.start L6.end
extrude "Выдавливание22" cut sketch "Эскиз30" against normal blind 3
sketch "Эскиз31" plane through (0, 3, 0) normal (0, 1, 0) x (1, 0, 0)
  line L0 (37, 203) -> (37, 31.5) projected
  line L1 (163, 31.5) -> (163, 203) projected
  line L2 (163, 117.25) -> (147.6, 117.25)
  line L3 (52.4, 117.25) -> (52.4, 94.9)
  line L4 (52.4, 94.9) -> (52.4, 139.6)
  line L5 (147.6, 117.25) -> (147.6, 139.6)
  line L6 (147.6, 139.6) -> (147.6, 94.9)
  line L7 (52.4, 94.9) -> (147.6, 94.9)
  line L8 (147.6, 94.9) -> (147.6, 139.6)
  line L9 (147.6, 139.6) -> (52.4, 139.6)
  line L10 (52.4, 139.6) -> (52.4, 94.9)
  line L11 (52.4, 117.25) -> (52.4, 80.5)
  line L12 (52.4, 80.5) -> (52.4, 154)
  line L13 (147.6, 117.25) -> (147.6, 154)
  line L14 (37, 80.5) -> (163, 80.5)
  line L15 (163, 80.5) -> (163, 154)
  line L16 (163, 154) -> (37, 154)
  line L17 (37, 154) -> (37, 80.5)
  line L18 (147.6, 94.9) -> (147.6, 80.5)
  line L19 (123.4115, 80.5) -> (123.4115, 154)
  circle A0 centre (139.7829, 87.7) radius 1.5
  circle A1 centre (156.3608, 92.8441) radius 1.5
  circle A2 centre (139.7829, 146.8) radius 1.5
  circle A3 centre (156.3608, 141.6559) radius 1.5
  line L20 (100, 80.5) -> (100, 154) construction
  circle A4 centre (60.2171, 87.7) radius 1.5
  circle A5 centre (43.6392, 92.8441) radius 1.5
  circle A6 centre (43.6392, 141.6559) radius 1.5
  circle A7 centre (60.2171, 146.8) radius 1.5
  point P0 (0, 0)
  point P1 (147.6, 139.6)
  point P2 (147.6, 139.6)
  dimension "d523" = 15.4
  dimension "d525" = 44.7
  dimension "d528" = 73.5
  dimension "d531" = 3
  constraints: 38 end point, 9 point on line, 8 centre point, 8 symmetric about line, 4 parallel, 3 horizontal, 3 midpoint, 3 perpendicular, 3 vertical, 1 collinear, 1 equal radius, 6 other
  measures "d523" distance of L2.start L2.end
  measures "d525" distance of L3.end L4.end
  measures "d528" distance of L11.end L12.end
  measures "d531" diameter of A0
ref_plane "РабПлоскость1" through (34, 0, -117.25) normal (0, 0, 1) x (1, 0, 0)
ref_plane "РабПлоскость2" through (100, 0, -203) normal (-1, 0, 0) x (0, 0, 1)
sketch "Эскиз32" plane through (0, 0, 0) normal (0, -1, 0) x (1, 0, 0)
  arc A0 (47.3111, -104.8304) -> (47.3111, -102.1696) centre (48.2, -103.5) ccw projected
  arc A1 (47.3111, -132.3304) -> (47.3111, -129.6696) centre (48.2, -131) ccw projected
  spline S0 degree 3 poles (47.3111, -132.3304) (47.2278, -132.2747) (47.1497, -132.2112) (46.9639, -132.0285) (46.8666, -131.8987) (46.7024, -131.5933) (46.6432, -131.4135) (46.5898, -131.0445) (46.5957, -130.8553) (46.6799, -130.4522) (46.7732, -130.2416) (47.0165, -129.9069) (47.1544, -129.7743) (47.3111, -129.6696) knots -0.981765 -0.981765 -0.981765 -0.981765 -0.793848 -0.793848 -0.49318 -0.49318 -0.143622 -0.143622 0.205938 0.205938 0.628487 0.628487 0.981765 0.981765 0.981765 0.981765 weights 1 1 1 1 1 1 1 1 1 1 1 1 1 1 projected
  spline S1 degree 3 poles (47.3111, -104.8304) (47.2278, -104.7747) (47.1497, -104.7112) (46.9639, -104.5285) (46.8666, -104.3987) (46.7024, -104.0933) (46.6432, -103.9135) (46.5898, -103.5445) (46.5957, -103.3553) (46.6799, -102.9522) (46.7732, -102.7416) (47.0165, -102.4069) (47.1544, -102.2743) (47.3111, -102.1696) knots -0.981765 -0.981765 -0.981765 -0.981765 -0.793848 -0.793848 -0.49318 -0.49318 -0.143622 -0.143622 0.205938 0.205938 0.628487 0.628487 0.981765 0.981765 0.981765 0.981765 weights 1 1 1 1 1 1 1 1 1 1 1 1 1 1 projected
  circle A2 centre (48.2, -103.5) radius 1.5
  circle A3 centre (48.2, -131) radius 1.5
  circle A4 centre (151.8, -103.5) radius 1.5
  circle A5 centre (151.8, -131) radius 1.5
  point P0 (0, 0)
  dimension "d535" = 3
  dimension "d536" = 3
  constraints: 4 centre point, 2 coincident
  measures "d535" diameter of A2
  measures "d536" diameter of A3
extrude "Выдавливание24" cut sketch "Эскиз32" against normal blind 10 contours A2 | A3 | A4 | A5
